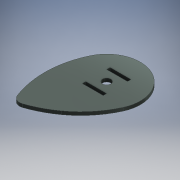
# Autodesk Inventor part: leva00
Saved by Autodesk Inventor 2016 (Build 200138000, 138)
## iProperties
Created: 2016-09-20
Part Number: leva00
Material: Madera (abedul)
Document SubType Name: Modeling
Designer: i95sa
Density: 0.55 g/cm^3
Appearance: Gris plomo - Pulido
Author: i95sa
Autodesk Inventor part; units mm, degrees
ref_plane "YZ Plane" through (0, 0, 0) normal (1, 0, 0) x (0, 1, 0)
ref_plane "XZ Plane" through (0, 0, 0) normal (0, 1, 0) x (-1, 0, 0)
ref_plane "XY Plane" through (0, 0, 0) normal (0, 0, 1) x (1, 0, 0)
sketch "Boceto1" plane through (0, 0, 0) normal (0, 0, 1) x (1, 0, 0)
  arc A0 (17.2143, 36.5822) -> (-17.2143, -36.5822) centre (0, 0) ccw
  arc A1 (-26.4914, -56.2971) -> (-34.4364, -73.1811) centre (-30.4639, -64.7391) ccw
  line L0 (-35.5866, -75.6253) -> (-44.0286, -71.6528)
  line L1 (-36.3757, 17.6464) -> (-50.4457, 24.2673)
  line L2 (-50.4457, 24.2673) -> (-44.0286, -71.6528)
  line L3 (-44.0286, -71.6528) -> (-46.5198, -34.416)
  arc A2 (-36.3757, 17.6464) -> (-46.5198, -34.416) centre (56.7082, -27.51) ccw
  arc A3 (-46.5198, -34.416) -> (-39.1875, -68.0477) centre (70.0479, -26.6176) ccw
  line L4 (1.3242, 2.814) -> (17.2143, 36.5822)
  line L5 (-1.3242, -2.814) -> (-35.5866, -75.6253)
  arc A4 (-17.2143, -36.5822) -> (17.2143, 36.5822) centre (0, 0) ccw
  arc A5 (-34.4364, -73.1811) -> (-26.4914, -56.2971) centre (-30.4639, -64.7391) ccw
  line L6 (-35.5866, -75.6253) -> (-27.1445, -79.5978)
  line L7 (36.7835, -16.7797) -> (50.8536, -23.4006)
  line L8 (50.8536, -23.4006) -> (-27.1445, -79.5978)
  line L9 (-27.1445, -79.5978) -> (3.1348, -57.7817)
  arc A6 (3.1348, -57.7817) -> (36.7835, -16.7797) centre (-57.344, 26.1589) ccw
  arc A7 (-27.4526, -73.5698) -> (3.1348, -57.7817) centre (-65.1594, 37.0062) ccw
  dimension "d0" = 80.86
  dimension "d6" = 18.66
  dimension "d7" = 9.33
  dimension "d8" = 15.55
  dimension "d9" = 37.32
  constraints: 20 end point, 20 point on circle, 8 centre point, 6 symmetric about line, 5 point on line, 4 tangent, 1 collinear, 4 other
  measures "d0" diameter of A0
  measures "d6" diameter of A1
  measures "d7" distance of L0.start L0.end
  measures "d8" distance of L1.start L1.end
  measures "d9" distance of L0.end L3.end
extrude "Extrusión2" add sketch "Boceto1" along normal blind 4 contours A4 A0 | A0 L5 A1 A3 A2 | A6 A7 A5 L5 A4 | L5 A1 | A5 L5
sketch "Boceto2" plane through (0, 0, 4) normal (0, 0, 1) x (1, 0, 0)
  line L0 (0, 0) -> (0, 12.5)
  line L1 (0, 12.5) -> (-12.5, 12.5)
  line L2 (-12.5, 12.5) -> (-12.5, 16.7)
  line L3 (-12.5, 16.7) -> (12.5, 16.7)
  line L4 (12.5, 16.7) -> (12.5, 12.5)
  line L5 (12.5, 12.5) -> (0, 12.5)
  line L6 (0, 0) -> (12.5, 0)
  line L7 (0, 0) -> (0, -12.5)
  line L8 (0, -12.5) -> (-12.5, -12.5)
  line L9 (-12.5, -12.5) -> (-12.5, -16.7)
  line L10 (-12.5, -16.7) -> (12.5, -16.7)
  line L11 (12.5, -16.7) -> (12.5, -12.5)
  line L12 (12.5, -12.5) -> (0, -12.5)
  circle A0 centre (0, 0) radius 5
  dimension "d24" = 12.5
  dimension "d25" = 12.5
  dimension "d26" = 4.2
  dimension "d27" = 25
  dimension "d28" = 10
  constraints: 26 end point, 5 perpendicular, 5 symmetric about line, 3 point on line, 1 centre point, 1 coincident, 1 parallel, 1 vertical
  measures "d24" distance of L0.start L0.end
  measures "d25" distance of L0.end L1.end
  measures "d26" distance of L1.end L2.end
  measures "d27" distance of L2.end L3.end
  measures "d28" diameter of A0
extrude "Extrusión3" cut sketch "Boceto2" against normal blind 4
